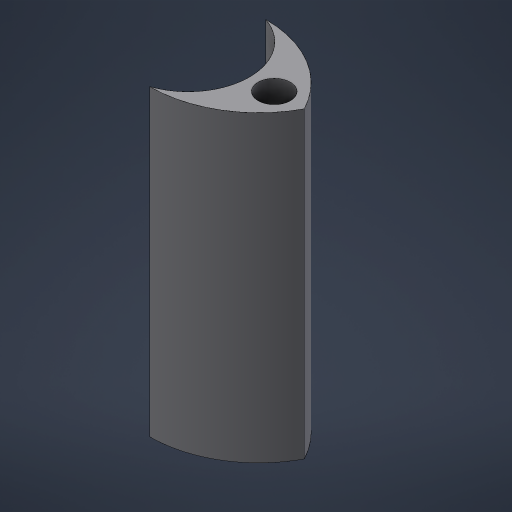
# Autodesk Inventor part: Abstandhalter_2
Saved by Autodesk Inventor 2023.5 (Build 275446000, 446)
## iProperties
Created: 2025-03-27
Part Number: Abstandhalter_2
Material: Generisch
Document SubType Name: Modeling
Designer: David Lill
Density: 1 g/cm^3
Appearance: Vorgabe
Author: David Lill
Autodesk Inventor part; units mm, degrees
ref_plane "YZ Plane" through (0, 0, 0) normal (1, 0, 0) x (0, 1, 0)
ref_plane "XZ Plane" through (0, 0, 0) normal (0, 1, 0) x (-1, 0, 0)
ref_plane "XY Plane" through (0, 0, 0) normal (0, 0, 1) x (1, 0, 0)
sketch "Skizze1" plane through (0, 0, 0) normal (0, 0, 1) x (1, 0, 0)
  arc A0 (0, 11.25) -> (-14.9586, 20.25) centre (-14.9586, 3.3189) ccw
  arc A1 (-14.9586, 2.25) -> (-14.9586, 20.25) centre (-18, 11.25) ccw
  arc A2 (-14.9586, 2.25) -> (0, 11.25) centre (-14.9586, 19.1811) ccw
  arc A3 (0, 78.75) -> (-14.9586, 87.75) centre (-14.9586, 70.8189) ccw
  arc A4 (-14.9586, 69.75) -> (-14.9586, 87.75) centre (-18, 78.75) ccw
  arc A5 (-14.9586, 69.75) -> (0, 78.75) centre (-14.9586, 86.6811) ccw
  line L0 (0, 0) -> (0, 270)
  line L1 (0, 270) -> (-4.65, 164)
  arc A6 (-4.65, 164) -> (-4.65, 156) centre (-4.65, 160) ccw
  line L2 (-4.65, 156) -> (0, 156)
  line L3 (0, 0) -> (0, 270)
  line L4 (0, 270) -> (-4.65, 219)
  arc A7 (-4.65, 219) -> (-4.65, 211) centre (-4.65, 215) ccw
  line L5 (-4.65, 211) -> (0, 211)
  line L6 (0, 135) -> (-167, 135)
  line L7 (-167, 135) -> (0, 270)
  line L8 (0, 270) -> (-167, 270)
  line L9 (-167, 270) -> (-167, 0)
  line L10 (-83.5, 270) -> (-83.5, 0)
  line L11 (-83.5, 0) -> (-167, 270)
  line L12 (-167, 270) -> (-167, 0)
  line L13 (-167, 0) -> (0, 0)
  line L14 (0, 0) -> (-167, 0)
  line L15 (-144.5, 31.5) -> (-165.5, 31.5)
  line L16 (-165.5, 31.5) -> (-165.5, 58.5)
  line L17 (-165.5, 58.5) -> (-144.5, 58.5)
  line L18 (-144.5, 58.5) -> (-144.5, 31.5)
  line L19 (-144.5, 238.5) -> (-165.5, 238.5)
  line L20 (-165.5, 238.5) -> (-165.5, 211.5)
  line L21 (-165.5, 211.5) -> (-144.5, 211.5)
  line L22 (-144.5, 211.5) -> (-144.5, 238.5)
  arc A8 (0, 258.75) -> (-14.9586, 267.75) centre (-14.9586, 250.8189) ccw
  arc A9 (-14.9586, 249.75) -> (0, 258.75) centre (-14.9586, 266.6811) ccw
  arc A10 (-14.9586, 249.75) -> (-14.9586, 267.75) centre (-18, 258.75) ccw
  arc A11 (0, 191.25) -> (-14.9586, 200.25) centre (-14.9586, 183.3189) ccw
  arc A12 (-14.9586, 182.25) -> (-14.9586, 200.25) centre (-18, 191.25) ccw
  arc A13 (-14.9586, 182.25) -> (0, 191.25) centre (-14.9586, 199.1811) ccw
  line L23 (-135.0414, 87.75) -> (-158, 87.75)
  arc A14 (-158, 87.75) -> (-158, 69.75) centre (-158, 78.75) ccw
  line L24 (-158, 69.75) -> (-135.0414, 69.75)
  arc A15 (-135.0414, 87.75) -> (-135.0414, 69.75) centre (-132, 78.75) ccw
  line L25 (-158, 182.25) -> (-135.0414, 182.25)
  arc A16 (-135.0414, 200.25) -> (-135.0414, 182.25) centre (-132, 191.25) ccw
  line L26 (-135.0414, 200.25) -> (-158, 200.25)
  arc A17 (-158, 200.25) -> (-158, 182.25) centre (-158, 191.25) ccw
  line L27 (-143, 0) -> (-143, 55)
  arc A18 (-143, 55) -> (-148, 60) centre (-148, 55) ccw
  line L28 (-148, 60) -> (-167, 60)
  line L29 (-167, 25) -> (-148, 25)
  arc A19 (-143, 20) -> (-148, 25) centre (-148, 20) ccw
  line L30 (-143, 270) -> (-143, 215)
  arc A20 (-148, 210) -> (-143, 215) centre (-148, 215) ccw
  line L31 (-148, 210) -> (-167, 210)
  line L32 (-167, 245) -> (-148, 245)
  arc A21 (-148, 245) -> (-143, 250) centre (-148, 250) ccw
  line L33 (0, 219) -> (-4.65, 219)
  arc A22 (-4.65, 219) -> (-4.65, 211) centre (-4.65, 215) ccw
  line L34 (-4.65, 211) -> (0, 211)
  line L35 (0, 164) -> (-4.65, 164)
  arc A23 (-4.65, 164) -> (-4.65, 156) centre (-4.65, 160) ccw
  line L36 (-4.65, 156) -> (0, 156)
  line L37 (-167, 156) -> (-162.35, 156)
  arc A24 (-162.35, 156) -> (-162.35, 164) centre (-162.35, 160) ccw
  line L38 (-162.35, 164) -> (-167, 164)
  line L39 (0, 59) -> (-4.65, 59)
  arc A25 (-4.65, 59) -> (-4.65, 51) centre (-4.65, 55) ccw
  line L40 (-4.65, 51) -> (0, 51)
  line L41 (0, 106) -> (-4.65, 106)
  arc A26 (-4.65, 114) -> (-4.65, 106) centre (-4.65, 110) ccw
  line L42 (-4.65, 114) -> (0, 114)
  line L43 (-167, 106) -> (-162.35, 106)
  arc A27 (-162.35, 106) -> (-162.35, 114) centre (-162.35, 110) ccw
  line L44 (-162.35, 114) -> (-167, 114)
  circle A28 centre (-18, 236.25) radius 9
  circle A29 centre (-18, 258.75) radius 9
  circle A30 centre (-18, 213.75) radius 9
  circle A31 centre (-18, 168.75) radius 9
  circle A32 centre (-18, 123.75) radius 9
  circle A33 centre (-18, 78.75) radius 9
  circle A34 centre (-18, 33.75) radius 9
  circle A35 centre (-18, 11.25) radius 9
  circle A36 centre (-18, 56.25) radius 9
  circle A37 centre (-18, 101.25) radius 9
  circle A38 centre (-18, 146.25) radius 9
  circle A39 centre (-18, 191.25) radius 9
  circle A40 centre (-37, 236.25) radius 9
  circle A41 centre (-37, 258.75) radius 9
  circle A42 centre (-37, 213.75) radius 9
  circle A43 centre (-37, 168.75) radius 9
  circle A44 centre (-37, 123.75) radius 9
  circle A45 centre (-37, 78.75) radius 9
  circle A46 centre (-37, 33.75) radius 9
  circle A47 centre (-37, 11.25) radius 9
  circle A48 centre (-37, 56.25) radius 9
  circle A49 centre (-37, 101.25) radius 9
  circle A50 centre (-37, 146.25) radius 9
  circle A51 centre (-37, 191.25) radius 9
  circle A52 centre (-56, 236.25) radius 9
  circle A53 centre (-56, 258.75) radius 9
  circle A54 centre (-56, 213.75) radius 9
  circle A55 centre (-56, 168.75) radius 9
  circle A56 centre (-56, 123.75) radius 9
  circle A57 centre (-56, 78.75) radius 9
  circle A58 centre (-56, 33.75) radius 9
  circle A59 centre (-56, 11.25) radius 9
  circle A60 centre (-56, 56.25) radius 9
  circle A61 centre (-56, 101.25) radius 9
  circle A62 centre (-56, 146.25) radius 9
  circle A63 centre (-56, 191.25) radius 9
  circle A64 centre (-75, 236.25) radius 9
  circle A65 centre (-75, 258.75) radius 9
  circle A66 centre (-75, 213.75) radius 9
  circle A67 centre (-75, 168.75) radius 9
  circle A68 centre (-75, 123.75) radius 9
  circle A69 centre (-75, 78.75) radius 9
  circle A70 centre (-75, 33.75) radius 9
  circle A71 centre (-75, 11.25) radius 9
  circle A72 centre (-75, 56.25) radius 9
  circle A73 centre (-75, 101.25) radius 9
  circle A74 centre (-75, 146.25) radius 9
  circle A75 centre (-75, 191.25) radius 9
  circle A76 centre (-94, 236.25) radius 9
  circle A77 centre (-94, 258.75) radius 9
  circle A78 centre (-94, 213.75) radius 9
  circle A79 centre (-94, 168.75) radius 9
  circle A80 centre (-94, 123.75) radius 9
  circle A81 centre (-94, 78.75) radius 9
  circle A82 centre (-94, 33.75) radius 9
  circle A83 centre (-94, 11.25) radius 9
  circle A84 centre (-94, 56.25) radius 9
  circle A85 centre (-94, 101.25) radius 9
  circle A86 centre (-94, 146.25) radius 9
  circle A87 centre (-94, 191.25) radius 9
  circle A88 centre (-113, 236.25) radius 9
  circle A89 centre (-113, 258.75) radius 9
  circle A90 centre (-113, 213.75) radius 9
  circle A91 centre (-113, 168.75) radius 9
  circle A92 centre (-113, 123.75) radius 9
  circle A93 centre (-113, 78.75) radius 9
  circle A94 centre (-113, 33.75) radius 9
  circle A95 centre (-113, 11.25) radius 9
  circle A96 centre (-113, 56.25) radius 9
  circle A97 centre (-113, 101.25) radius 9
  circle A98 centre (-113, 146.25) radius 9
  circle A99 centre (-113, 191.25) radius 9
  circle A100 centre (-132, 236.25) radius 9
  circle A101 centre (-132, 191.25) radius 9
  circle A102 centre (-132, 146.25) radius 9
  circle A103 centre (-132, 101.25) radius 9
  circle A104 centre (-132, 56.25) radius 9
  circle A105 centre (-132, 11.25) radius 9
  circle A106 centre (-132, 33.75) radius 9
  circle A107 centre (-132, 78.75) radius 9
  circle A108 centre (-132, 123.75) radius 9
  circle A109 centre (-132, 168.75) radius 9
  circle A110 centre (-132, 213.75) radius 9
  circle A111 centre (-132, 258.75) radius 9
  line L45 (0, 0) -> (0, 270)
  line L46 (-167, 0) -> (0, 0)
  line L47 (-167, 270) -> (-167, 0)
  line L48 (-167, 0) -> (0, 0)
  line L49 (0, 270) -> (-167, 270)
  line L50 (0, 135) -> (-167, 135)
  line L51 (-14.9586, 2.25) -> (-18, 2.25)
  circle A112 centre (-18, 11.25) radius 9
  circle A113 centre (-4.65, 11.25) radius 2.5
  circle A114 centre (-4.65, 78.75) radius 2.5
  circle A115 centre (-4.65, 191.25) radius 2.5
  circle A116 centre (-4.65, 258.75) radius 2.5
  circle A117 centre (-162.35, 78.75) radius 2.5
  circle A118 centre (-162.35, 191.25) radius 2.5
  circle A119 centre (-151, 78.75) radius 7
  circle A120 centre (-151, 191.25) radius 7
  line L52 (-83.5, 270) -> (-83.5, 0)
  point P0 (0, 78.75)
  constraints: 121 centre point, 106 end point, 56 point on circle
extrude "Extrusion1" add sketch "Skizze1" along normal blind 47 contours A5 A4 A3
